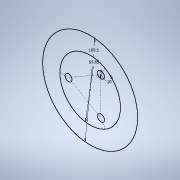
# Autodesk Inventor part: Tractor_Static_2
Saved by Autodesk Inventor 2022 (Build 260153070, 153G)
## iProperties
Created: 2022-03-05
Part Number: Tractor_Static_2
Material: Generic
Document SubType Name: Modeling
Designer: a laptop
Density: 1 g/cm^3
Appearance: Default
Author: a laptop
Autodesk Inventor part; units mm, degrees
ref_plane "YZ Plane" through (0, 0, 0) normal (1, 0, 0) x (0, 1, 0)
ref_plane "XZ Plane" through (0, 0, 0) normal (0, 1, 0) x (-1, 0, 0)
ref_plane "XY Plane" through (0, 0, 0) normal (0, 0, 1) x (1, 0, 0)
sketch "Sketch1" plane through (0, 0, 0) normal (0, 0, 1) x (1, 0, 0)
  circle A0 centre (0, 0) radius 34.925 construction
  circle A1 centre (0, 0) radius 54.75
  circle A2 centre (12.4625, 21.5857) radius 4
  circle A3 centre (-24.925, 0) radius 4
  circle A4 centre (12.4625, -21.5857) radius 4
  line L0 (-24.925, 0) -> (12.4625, 21.5857) construction
  line L1 (12.4625, 21.5857) -> (12.4625, -21.5857) construction
  line L2 (12.4625, -21.5857) -> (-24.925, 0) construction
  line L3 (12.4625, 21.5857) -> (17.4625, 30.2459) construction
  line L4 (12.4625, -21.5857) -> (17.4625, -30.2459) construction
  line L5 (-24.925, 0) -> (-34.925, 0) construction
  circle A5 centre (0, 0) radius 10
  dimension "d0" = 69.85
  dimension "d1" = 109.5
  dimension "d2" = 8
  dimension "d3" = 10
  dimension "d4" = 20
  constraints: 12 end point, 6 centre point, 4 equal length, 3 coincident, 3 line through centre, 3 point on circle, 2 equal radius, 1 horizontal
  measures "d0" diameter of A0
  measures "d1" diameter of A1
  measures "d2" diameter of A2
  measures "d3" distance of L0.end L3.end
  measures "d4" diameter of A5
extrude "Extrusion1" add sketch "Sketch1" along normal blind 10
sketch "Sketch2" plane through (0, 0, 10) normal (0, 0, 1) x (1, 0, 0)
  circle A0 centre (0, 0) radius 10 projected
  line L0 (-2.5, 9.5) -> (2.5, 9.5)
  line L1 (2.5, 9.5) -> (2.5, 8)
  line L2 (2.5, 8) -> (-2.5, 8)
  line L3 (-2.5, 8) -> (-2.5, 9.5)
  line L4 (-2.5, -8) -> (2.5, -8)
  line L5 (2.5, -8) -> (2.5, -9.5)
  line L6 (2.5, -9.5) -> (-2.5, -9.5)
  line L7 (-2.5, -9.5) -> (-2.5, -8)
  line L8 (-2.5, 8) -> (0, 0) construction
  line L9 (0, 0) -> (2.5, 8) construction
  line L10 (0, 0) -> (-2.5, -8) construction
  line L11 (2.5, -8) -> (0, 0) construction
  circle A1 centre (0, 6) radius 1.5
  circle A2 centre (0, -6) radius 1.5
  line L12 (0, -6) -> (0, 6) construction
  dimension "d7" = 5
  dimension "d8" = 1.5
  dimension "d10" = 8
  dimension "d13" = 3
  dimension "d15" = 12
  constraints: 26 end point, 6 equal length, 2 centre point, 2 collinear, 2 horizontal, 2 perpendicular, 1 coincident, 1 equal radius, 1 midpoint, 1 point on line, 1 vertical
  measures "d7" distance of L0.start L0.end
  measures "d8" distance of L0.end L1.end
  measures "d10" distance from line of point (0, 0) L2
  measures "d13" diameter of A1
  measures "d15" distance of L12.start L12.end
extrude "Extrusion2" add sketch "Sketch2" against normal blind 5
body "Solid1"
